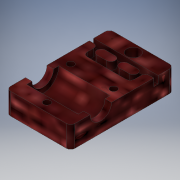
# Autodesk Inventor part: Lagerblock XY
Saved by Autodesk Inventor 2018.2 (Build 222227000, 227)
## iProperties
Part Number: Lagerblock XY
Material: ABS-Kunststoff
Document SubType Name: Modeling
Designer: Till
Density: 1.06 g/cm^3
Appearance: Rot
Author: Till
Autodesk Inventor part; units mm, degrees
ref_plane "YZ Plane" through (0, 0, 0) normal (1, 0, 0) x (0, 1, 0)
ref_plane "XZ Plane" through (0, 0, 0) normal (0, 1, 0) x (-1, 0, 0)
ref_plane "XY Plane" through (0, 0, 0) normal (0, 0, 1) x (1, 0, 0)
sketch "Skizze3" plane through (0, 0, 0) normal (0, 0, 1) x (1, 0, 0)
  line L0 (0, 0) -> (30, 0)
  line L1 (30, 0) -> (30, 48)
  line L2 (30, 48) -> (0, 48)
  line L3 (0, 48) -> (0, 0)
  dimension "d14" = 30
  dimension "d15" = 48
  constraints: 8 end point, 2 parallel, 1 horizontal, 1 perpendicular
  measures "d14" distance of L2.end L1.end
  measures "d15" distance of L1.end L0.end
extrude "Extrusion3" add sketch "Skizze3" along normal blind 10
sketch "Skizze4" plane through (0, 0, 0) normal (-1, 0, 0) x (0, 0, 1)
  line L0 (10, 0) -> (10, 48) projected
  arc A0 (10, 21.5) -> (10, 6.5) centre (10, 14) ccw
  line L1 (10, 21.5) -> (10, 6.5)
  point P0 (0, 0)
  dimension "d18" = 7.5
  dimension "d19" = 14
  constraints: 2 end point, 2 point on circle, 2 point on line, 1 centre point, 1 collinear
  measures "d18" radius of A0
  measures "d19" distance of L0.start A0.centre
extrude "Extrusion4" cut sketch "Skizze4" against normal up to next
sketch "Skizze5" plane through (0, 0, 10) normal (0, 0, 1) x (1, 0, 0)
  line L0 (0, 40.7) -> (30, 40.7)
  line L1 (30, 40.7) -> (30, 38.7)
  line L2 (0, 38.7) -> (0, 40.7)
  line L3 (30, 38.7) -> (28, 38.7)
  line L4 (0, 38.7) -> (2, 38.7)
  line L5 (30, 48) -> (0, 48) projected
  line L6 (26, 36.7) -> (26, 33.7)
  line L7 (24, 31.7) -> (6, 31.7)
  line L8 (4, 33.7) -> (4, 36.7)
  line L9 (0, 21.5) -> (30, 21.5) projected
  arc A0 (4, 36.7) -> (2, 38.7) centre (2, 36.7) ccw
  arc A1 (4, 33.7) -> (6, 31.7) centre (6, 33.7) ccw
  arc A2 (24, 31.7) -> (26, 33.7) centre (24, 33.7) ccw
  arc A3 (28, 38.7) -> (26, 36.7) centre (28, 36.7) ccw
  line L10 (7.5, 36.7) -> (12, 36.7) construction
  line L11 (7.5, 34.7) -> (12, 34.7)
  line L12 (12, 38.7) -> (7.5, 38.7)
  arc A4 (7.5, 38.7) -> (7.5, 34.7) centre (7.5, 36.7) ccw
  arc A5 (12, 34.7) -> (12, 38.7) centre (12, 36.7) ccw
  line L13 (18, 36.7) -> (22.5, 36.7) construction
  line L14 (18, 34.7) -> (22.5, 34.7)
  line L15 (22.5, 38.7) -> (18, 38.7)
  arc A6 (18, 38.7) -> (18, 34.7) centre (18, 36.7) ccw
  arc A7 (22.5, 34.7) -> (22.5, 38.7) centre (22.5, 36.7) ccw
  line L16 (30, 21.5) -> (30, 48) projected
  line L17 (0, 48) -> (0, 21.5) projected
  point P0 (26, 38.7)
  point P1 (4, 38.7)
  point P2 (26, 31.7)
  point P3 (4, 31.7)
  point P4 (9.75, 36.7)
  point P5 (20.25, 36.7)
  dimension "d22" = 2
  dimension "d28" = 4
  dimension "d29" = 4
  dimension "d30" = 2
  dimension "d34" = 7
  dimension "d48" = 2
  dimension "d83" = 7.3
  dimension "d84" = 4.5
  dimension "d85" = 4
  dimension "d86" = 3.5
  dimension "d87" = 5
  dimension "d88" = 4.5
  dimension "d89" = 4
  dimension "d90" = 3.5
  dimension "d91" = 5
  constraints: 32 end point, 16 point on circle, 16 tangent, 8 centre point, 8 point on line, 4 perpendicular, 3 equal radius, 3 horizontal, 3 parallel, 2 collinear, 2 midpoint, 1 vertical
  measures "d22" distance of L0.end L1.end
  measures "d28" distance of L1.end point (26, 38.7)
  measures "d29" distance of L2.start point (4, 38.7)
  measures "d30" distance between parallel lines of L0 L4
  measures "d34" distance of point (26, 38.7) point (26, 31.7)
  measures "d48" radius of A0
  measures "d83" distance between parallel lines of L5 L0
  measures "d84" distance of L10.start L10.end
  measures "d85" diameter of A5
  measures "d86" distance from line of L8 L10.start
  measures "d87" distance from line of L7 point (9.75, 36.7)
  measures "d88" distance of L13.start L13.end
  measures "d89" diameter of A7
  measures "d90" distance from line of L6 L13.end
  measures "d91" distance from line of L7 point (20.25, 36.7)
extrude "Extrusion5" cut sketch "Skizze5" against normal blind 3.5 contours L0 L1 L3 A3 L6 A2 L7 A1 L8 A0 L4 L2
sketch "Skizze6" plane through (0, 0, 10) normal (0, 0, 1) x (1, 0, 0)
  line L0 (0, 48) -> (0, 0) projected
  line L1 (30, 0) -> (30, 48) projected
  circle A0 centre (15, 44.2) radius 3.05
  line L2 (0, 40.7) -> (30, 40.7) projected
  dimension "d43" = 6.1
  dimension "d44" = 15
  dimension "d45" = 3.5
  constraints: 1 centre point
  measures "d43" diameter of A0
  measures "d44" distance from line of L1 A0.centre
  measures "d45" distance from line of L2 A0.centre
extrude "Extrusion6" cut sketch "Skizze6" against normal up to next
sketch "Skizze7" plane through (0, 0, 10) normal (0, 0, 1) x (1, 0, 0)
  circle A0 centre (5, 25) radius 1.55
  circle A1 centre (25, 25) radius 1.55
  circle A2 centre (15, 4) radius 1.55
  line L0 (0, 6.5) -> (0, 21.5) projected
  line L1 (30, 21.5) -> (30, 6.5) projected
  line L2 (0, 0) -> (30, 0) projected
  line L3 (0, 6.5) -> (0, 0) projected
  line L4 (0, 21.5) -> (30, 21.5) projected
  point P0 (0, 38.7)
  point P1 (30, 38.7)
  dimension "d49" = 3.1
  dimension "d50" = 3.1
  dimension "d51" = 3.1
  dimension "d53" = 5
  dimension "d54" = 5
  dimension "d55" = 4
  dimension "d74" = 15
  dimension "d75" = 3.5
  dimension "d76" = 3.5
  constraints: 3 centre point
  measures "d49" diameter of A0
  measures "d50" diameter of A1
  measures "d51" diameter of A2
  measures "d53" distance from line of L0 A0.centre
  measures "d54" distance from line of L1 A1.centre
  measures "d55" distance from line of L2 A2.centre
  measures "d74" distance from line of L3 A2.centre
  measures "d75" distance from line of L4 A0.centre
  measures "d76" distance from line of L4 A1.centre
extrude "Extrusion7" cut sketch "Skizze7" against normal up to next
sketch "Skizze8" plane through (30, 0, 0) normal (1, 0, 0) x (0, 0, -1)
  arc A0 (-10, 6.5) -> (-10, 21.5) centre (-10, 14) ccw projected
  arc A1 (-10, 9) -> (-10, 19) centre (-10, 14) ccw
  line L0 (-10, 19) -> (-10, 21.5)
  line L1 (-10, 9) -> (-10, 6.5)
  arc A2 (-10, 6.5) -> (-10, 21.5) centre (-10, 14) ccw
  point P0 (0, 0)
  dimension "d59" = 5
  constraints: 4 end point, 4 point on circle, 2 centre point, 2 coincident, 1 collinear
  measures "d59" radius of A1
extrude "Extrusion8" add sketch "Skizze8" against normal blind 3
sketch "Skizze10" plane through (0, 0, 0) normal (-1, 0, 0) x (0, 0, 1)
  arc A0 (10, 19) -> (10, 9) centre (10, 14) ccw
  arc A1 (10, 21.5121) -> (10, 6.4879) centre (10, 14) ccw
  arc A2 (10, 19) -> (10, 9) centre (10, 14) ccw projected
  line L0 (10, 19) -> (10, 21.5121)
  line L1 (10, 6.5) -> (10, 21.5) projected
  line L2 (10, 9) -> (10, 6.4879)
  point P0 (0, 0)
  point P1 (10, 38.7)
  constraints: 4 end point, 4 point on circle, 2 centre point, 1 coincident, 1 collinear
extrude "Extrusion9" add sketch "Skizze10" against normal blind 3 contours A0 L1 L2 A1 L0
fillet "Rundung1" radius 2 4 edges at (30, 0, 5) (0, 0, 5) (0, 48, 5) (30, 48, 5)
sketch "Skizze14" plane through (0, 0, 0) normal (0, 0, -1) x (-1, 0, 0)
  circle A0 centre (-5, 25) radius 1.55 projected
  circle A1 centre (-5, 25) radius 2.9 construction
  circle A2 centre (-25, 25) radius 1.55 projected
  circle A3 centre (-25, 25) radius 2.9 construction
  line L0 (-7.9, 26.6743) -> (-5, 28.3486)
  line L1 (-5, 28.3486) -> (-2.1, 26.6743)
  line L2 (-2.1, 26.6743) -> (-2.1, 23.3257)
  line L3 (-2.1, 23.3257) -> (-5, 21.6514)
  line L4 (-5, 21.6514) -> (-7.9, 23.3257)
  line L5 (-7.9, 23.3257) -> (-7.9, 26.6743)
  line L6 (-22.1, 23.3257) -> (-25, 21.6514)
  line L7 (-25, 21.6514) -> (-27.9, 23.3257)
  line L8 (-27.9, 23.3257) -> (-27.9, 26.6743)
  line L9 (-27.9, 26.6743) -> (-25, 28.3486)
  line L10 (-25, 28.3486) -> (-22.1, 26.6743)
  line L11 (-22.1, 26.6743) -> (-22.1, 23.3257)
  circle A4 centre (-15, 4) radius 2.9 construction
  line L12 (-16.6743, 1.1) -> (-18.3486, 4)
  line L13 (-18.3486, 4) -> (-16.6743, 6.9)
  line L14 (-16.6743, 6.9) -> (-13.3257, 6.9)
  line L15 (-13.3257, 6.9) -> (-11.6514, 4)
  line L16 (-11.6514, 4) -> (-13.3257, 1.1)
  line L17 (-13.3257, 1.1) -> (-16.6743, 1.1)
  point P0 (0, 0)
  point P1 (-7.9, 25)
  point P2 (-22.1, 25)
  point P3 (-15, 1.1)
  dimension "d92" = 5.8
  dimension "d95" = 5.8
  dimension "d98" = 5.8
  dimension "d99" = 0
  dimension "d100" = 0
  constraints: 36 end point, 6 coincident, 3 midpoint, 2 horizontal alignment, 1 vertical alignment, 45 other
  measures "d99" vertical distance of point (-7.9, 25) point (-5, 25)
  measures "d100" vertical distance of point (-25, 25) point (-22.1, 25)
extrude "Extrusion13" cut sketch "Skizze14" against normal blind 3.2
